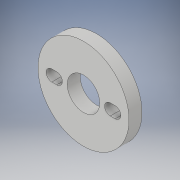
# Autodesk Inventor part: motormount
Saved by Autodesk Inventor 2019 (Build 230136000, 136)
## iProperties
Created: 2019-10-24
Part Number: motormount
Material: Generic
Document SubType Name: Modeling
Designer: robgr
Density: 1 g/cm^3
Appearance: Default
Author: robgr
Autodesk Inventor part; units mm, degrees
ref_plane "YZ Plane" through (0, 0, 0) normal (1, 0, 0) x (0, 1, 0)
ref_plane "XZ Plane" through (0, 0, 0) normal (0, 1, 0) x (-1, 0, 0)
ref_plane "XY Plane" through (0, 0, 0) normal (0, 0, 1) x (1, 0, 0)
sketch "Sketch1" plane through (0, 0, 0) normal (0, 0, 1) x (1, 0, 0)
  circle A0 centre (0, 0) radius 14
  dimension "d0" = 28
  constraints: 1 centre point, 1 coincident
  measures "d0" diameter of A0
extrude "Extrusion1" add sketch "Sketch1" along normal blind 4
sketch "Sketch2" plane through (0, 0, 4) normal (0, 0, 1) x (1, 0, 0)
  circle A0 centre (0, 0) radius 5
  line L0 (-11.5, 0) -> (-6.5, 0) construction
  line L1 (-9.75, -1.75) -> (-8.25, -1.75)
  line L2 (-8.25, 1.75) -> (-9.75, 1.75)
  arc A1 (-9.75, 1.75) -> (-9.75, -1.75) centre (-9.75, 0) ccw
  arc A2 (-8.25, -1.75) -> (-8.25, 1.75) centre (-8.25, 0) ccw
  line L3 (6.5, -0.0526) -> (11.5, -0.0526) construction
  line L4 (8.25, 1.6974) -> (9.75, 1.6974)
  line L5 (9.75, -1.8026) -> (8.25, -1.8026)
  arc A3 (8.25, 1.6974) -> (8.25, -1.8026) centre (8.25, -0.0526) ccw
  arc A4 (9.75, -1.8026) -> (9.75, 1.6974) centre (9.75, -0.0526) ccw
  point P0 (-9, 0)
  point P1 (9, -0.0526)
  dimension "d3" = 10
  dimension "d4" = 5
  dimension "d5" = 3.5
  dimension "d6" = 6.5
  dimension "d7" = 5
  dimension "d11" = 6.5
  dimension "d12" = 1.5
  constraints: 16 end point, 12 point on circle, 8 tangent, 5 centre point, 4 point on line, 2 horizontal, 2 midpoint, 2 parallel, 1 coincident
  measures "d3" diameter of A0
  measures "d4" distance of L0.start L0.end
  measures "d5" diameter of A2
  measures "d6" distance of A0.centre L0.end
  measures "d7" distance of L3.start L3.end
  measures "d11" horizontal distance of A0.centre L3.start
  measures "d12" distance of A4.centre A3.centre
extrude "Extrusion2" cut sketch "Sketch2" against normal blind 5
body "Solid1"
